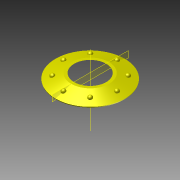
# Autodesk Inventor part: Small Suction Cup Part 2 1764
Saved by Autodesk Inventor 2011 (Build 150239000, 239)
## iProperties
Created: 2011-01-15
Part Number: Small Suction Cup Part 2 1764
Document SubType Name: Modeling
Designer: dfranz
Density: 1 g/cm^3
Author: dfranz
Autodesk Inventor part; units mm, degrees
ref_plane "XZ Plane" through (0, 0, 0) normal (0, 1, 0) x (-1, 0, 0)
ref_plane "XY Plane" through (0, 0, 0) normal (0, 0, 1) x (1, 0, 0)
sketch "Sketch1" plane through (0, 0, 0) normal (0, 0, 1) x (1, 0, 0)
  line L0 (7.377611, 14.798946) -> (-3.233216, 11.453365)
  line L1 (5.699167, 14.798946) -> (-3.384987, 11.934724)
  line L2 (-3.233216, 11.453365) -> (-3.384987, 11.934724)
  line L3 (7.377611, 14.798946) -> (5.699167, 14.798946)
  line L4 (16.623211, 19.826225) -> (16.623211, 7.345972)
  point P0 (0, 0)
  dimension "d0" = 1.67844
  dimension "d1" = 9.525
  dimension "d2" = 9.2456
  constraints: 10 end point, 1 perpendicular
  measures "d0" distance of L0.start L1.start
  measures "d1" distance of L1.start L2.end
  measures "d2" distance from line of L4 L0.start
revolve "Revolution1" add sketch "Sketch1" angle 360 about axis through (16.623211, 19.826225, 0) along (0, -1, 0)
ref_plane "Work Plane2" through (16.623211, 14.798946, 0) normal (1, 0, 0) x (0, 1, 0)
sketch "Sketch3" plane through (16.623211, 14.798946, 0) normal (1, 0, 0) x (0, 1, 0)
  line L0 (-2.864223, -20.008199) -> (0, -10.924045)
  line L1 (-1.432111, -15.466122) -> (2.15205, -16.596203)
  arc A0 (-1.814008, -16.677342) -> (-0.220891, -15.848018) centre (-1.432111, -15.466122) ccw
  point P0 (-14.798946, 0)
  dimension "d6" = 0
  dimension "d7" = 0
  dimension "d8" = 1.27
  constraints: 2 end point, 2 point on circle, 2 point on line, 1 centre point, 1 midpoint, 1 perpendicular
  measures "d6" distance from line of L0 A0.centre
  measures "d7" distance from line of L1 A0.centre
  measures "d8" distance of A0.start L1.start
revolve "Revolution2" add sketch "Sketch3" angle 360 about axis through (16.623211, 13.366835, -15.466122) along (0, 0.953717, -0.3007058)
pattern_circular "Circular Pattern1" count 8 over 360 about axis through (16.623211, 13.366835, 0) along (0, 1, 0) of "Revolution2"
body "Solid1"
